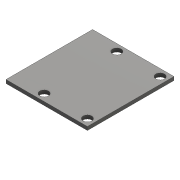
# Autodesk Inventor part: camerapi
Saved by Autodesk Inventor 2016 (Build 200138000, 138)
## iProperties
Created: 2015-12-16
Part Number: camerapi
Material: 一般
Document SubType Name: Modeling
Designer: NN
Density: 1 g/cm^3
Appearance: 滑らか - 黒
Mass: 0.868044 g
Surface Area: 14.1571 cm^2
Volume: 0.868044 cm^3
Author: NN
Autodesk Inventor part; units mm, degrees
ref_plane "YZ Plane" through (0, 0, 0) normal (1, 0, 0) x (0, 1, 0)
ref_plane "XZ Plane" through (0, 0, 0) normal (0, 1, 0) x (-1, 0, 0)
ref_plane "XY Plane" through (0, 0, 0) normal (0, 0, 1) x (1, 0, 0)
sketch "スケッチ1" plane through (0, 0, 0) normal (0, 0, 1) x (1, 0, 0)
  circle A0 centre (14.5, 10.5) radius 1.25
  circle A1 centre (14.5, -10.5) radius 1.25
  circle A2 centre (2, -10.5) radius 1.25
  circle A3 centre (2, 10.5) radius 1.25
  circle A4 centre (2.5, 0) radius 7
  line L0 (16.5, 12.5) -> (16.5, -12.5)
  line L1 (16.5, -12.5) -> (-7, -12.5)
  line L2 (-7, -12.5) -> (-7, 12.5)
  line L3 (-7, 12.5) -> (16.5, 12.5)
  circle A5 centre (2.5, 0) radius 7 projected
  circle A6 centre (2, -10.5) radius 2.5 projected
  circle A7 centre (2, 10.5) radius 2.5 projected
  circle A8 centre (14.5, 10.5) radius 2.5 projected
  circle A9 centre (14.5, -10.5) radius 2.5 projected
  point P0 (0, 0)
  dimension "d0" = 2.5
  dimension "d1" = 2.5
  dimension "d2" = 2.5
  dimension "d3" = 2.5
  dimension "d4" = 2
  dimension "d5" = 2
  dimension "d6" = 2
  dimension "d7" = 9
  constraints: 8 end point, 5 centre point, 4 concentric, 3 perpendicular, 1 vertical
  measures "d0" diameter of A0
  measures "d1" diameter of A1
  measures "d2" diameter of A3
  measures "d3" diameter of A2
  measures "d4" distance from line of A0.centre L0
  measures "d5" distance from line of L3 A0.centre
  measures "d6" distance from line of L1 A1.centre
  measures "d7" distance from line of L2 A2.centre
extrude "押し出し1" add sketch "スケッチ1" along normal blind 1 contours A4 | L0 A8 L3 | L0 A8 L3 | L0 A9 L1 A6 L2 L3 A7 A8 | L0 A9 L1 | A7 L3 | L0 L1 A9 | L1 A6 picked at (2.0502, 12.247) picked at (2.0502, -12.247)
sketch "スケッチ2" plane through (0, 0, 0) normal (0, 0, -1) x (-1, 0, 0)
  circle A0 centre (-2, 10.5) radius 1.25 projected
  circle A1 centre (-14.5, -10.5) radius 1.25 projected
  circle A2 centre (-2, -10.5) radius 1.25 projected
  circle A3 centre (-14.5, 10.5) radius 1.25 projected
  circle A4 centre (-2.5, 0) radius 7 projected
  line L0 (17.5, -15.5) -> (-17.5, -15.5) projected
  line L1 (-17.5, 15.5) -> (-17.5, -15.5) projected
  line L2 (-17.5, 15.5) -> (17.5, 15.5) projected
  line L3 (17.5, -15.5) -> (17.5, 15.5) projected
  line L4 (-6.5, 4) -> (1.5, 4)
  line L5 (1.5, 4) -> (1.5, -4)
  line L6 (1.5, -4) -> (-6.5, -4)
  line L7 (-6.5, -4) -> (-6.5, 4)
  line L8 (-6.5, 4) -> (1.5, -4) construction
  line L9 (1.5, 4) -> (-6.5, -4) construction
  point P0 (0, 0)
  dimension "d10" = 8
  dimension "d11" = 8
  constraints: 12 end point, 2 midpoint, 2 parallel, 1 horizontal, 1 perpendicular
  measures "d10" distance between parallel lines of L5 L7
  measures "d11" distance between parallel lines of L6 L4
extrude "押し出し2" add sketch "スケッチ2" along normal blind 4 contours L4 L5 L6 L7
sketch "スケッチ3" plane through (0, 0, -4) normal (0, 0, -1) x (-1, 0, 0)
  circle A0 centre (-2.5, 0) radius 7 projected
  circle A1 centre (-2.5, 0) radius 3.75
  point P0 (0, 0)
  dimension "d14" = 7.5
  constraints: 1 centre point, 1 coincident
  measures "d14" diameter of A1
extrude "押し出し3" add sketch "スケッチ3" along normal blind 1 contours A1
